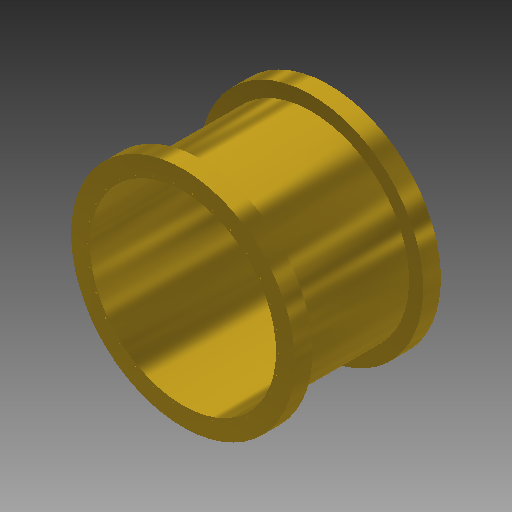
# Autodesk Inventor part: Electrode 5_6_7
Saved by Autodesk Inventor 2017 (Build 210142000, 142)
## iProperties
Created: 2009-05-06
Part Number: Electrode 5_6_7
Document SubType Name: Modeling
Designer: Serena
Material: Default
Density: 1 g/cm^3
Appearance: Glossy - Gold
Author: Serena
Autodesk Inventor part; units mm, degrees
ref_plane "YZ Plane" through (0, 0, 0) normal (1, 0, 0) x (0, 1, 0)
ref_plane "XZ Plane" through (0, 0, 0) normal (0, 1, 0) x (-1, 0, 0)
ref_plane "XY Plane" through (0, 0, 0) normal (0, 0, 1) x (1, 0, 0)
sketch "Sketch1" plane through (0, 0, 0) normal (0, 0, 1) x (1, 0, 0)
  circle A0 centre (0, 0) radius 100.35
  circle A1 centre (0, 0) radius 105.35
  dimension "d0" = 200.7
  dimension "d1" = 210.7
  constraints: 2 centre point, 1 coincident
  measures "d0" diameter of A0
  measures "d1" diameter of A1
extrude "Extrusion1" add sketch "Sketch1" along normal blind 157.48
sketch "Sketch3" plane through (0, 0, 0) normal (0, 1, 0) x (-1, 0, 0)
  line L0 (-105.35, 157.48) -> (105.35, 157.48) projected
  line L1 (-105.35, 0) -> (105.35, 0) projected
  line L2 (100.35, 0) -> (100.35, 157.48) projected
  line L3 (105.35, 0) -> (105.35, 157.48) projected
  line L4 (102.85, 157.48) -> (102.85, 55.0181)
  line L5 (102.85, 143.2846) -> (100.35, 143.2846)
  line L6 (102.85, 140.5603) -> (105.35, 140.5603)
  line L7 (102.85, 157.48) -> (102.85, 158.3207)
  circle A0 centre (102.85, 157.98) radius 1
  line L8 (102.85, 157.48) -> (102.85, 156.98)
  line L9 (102.85, 157.48) -> (103.716, 157.48)
  arc A1 (102.85, 156.98) -> (103.716, 157.48) centre (102.85, 157.98) ccw
  line L10 (102.85, 157.48) -> (102.85, 156.98)
  line L11 (102.85, 157.48) -> (103.716, 157.48)
  arc A2 (102.85, 156.98) -> (103.716, 157.48) centre (102.85, 157.98) ccw
  line L12 (102.85, 157.48) -> (102.85, 156.98)
  line L13 (102.85, 157.48) -> (101.984, 157.48)
  arc A3 (101.984, 157.48) -> (102.85, 156.98) centre (102.85, 157.98) ccw
  dimension "d15" = 2
  dimension "d16" = 0.5
  constraints: 20 end point, 9 point on circle, 9 point on line, 5 concentric, 4 centre point, 3 collinear, 3 perpendicular, 2 parallel
  measures "d15" diameter of A0
  measures "d16" distance of L4.start L8.end
revolve "Revolution1" cut sketch "Sketch3" angle 360 about axis through (-102.85, 0, 157.48) along (0, 0, -1) picked at (102.3136, 157.4236) contours L0 L4 A0
pattern_circular "Circular Pattern1" count 30 over 360 about axis through (0, 0, 0) along (0, 0, 1) of "Revolution1"
sketch "Sketch4" plane through (0, 0, 0) normal (0, 1, 0) x (-1, 0, 0)
  line L0 (-100.35, 157.48) -> (100.35, 157.48) projected
  line L1 (100.35, 0) -> (-100.35, 0) projected
  line L2 (105.35, 0) -> (105.35, 157.48) projected
  line L3 (-105.35, 0) -> (105.35, 0) projected
  line L4 (100.35, 0) -> (100.35, 157.48) projected
  line L5 (102.85, 0) -> (102.85, 39.0845)
  line L6 (102.85, 39.0845) -> (102.85, 4.4381)
  line L7 (100.35, 4.4381) -> (102.85, 4.4381)
  line L8 (102.85, 5.9556) -> (105.35, 5.9556)
  line L9 (102.85, 0) -> (102.85, -6.1846)
  circle A0 centre (102.85, -0.5) radius 1
  line L10 (102.85, 0.5) -> (102.85, 0)
  line L11 (102.85, 0) -> (103.716, 0)
  line L12 (102.85, 0) -> (101.984, 0)
  arc A1 (102.85, 0.5) -> (101.984, 0) centre (102.85, -0.5) ccw
  arc A2 (103.716, 0) -> (102.85, 0.5) centre (102.85, -0.5) ccw
  dimension "d21" = 2
  dimension "d22" = 0.5
  constraints: 16 end point, 9 point on line, 7 point on circle, 3 centre point, 3 concentric, 3 perpendicular, 2 parallel, 1 collinear
  measures "d21" diameter of A0
  measures "d22" distance of L10.start L5.start
revolve "Revolution2" cut sketch "Sketch4" angle 360 about axis through (-102.85, 0, 0.5) along (0, 0, -1) picked at (102.3136, 0.0564) contours L3 A0 L5
pattern_circular "Circular Pattern2" count 30 over 360 about axis through (0, 0, 0) along (0, 0, 1) of "Revolution2"
sketch "Sketch5" plane through (0, 0, 157.48) normal (0, 0, 1) x (1, 0, 0)
  circle A0 centre (0, 0) radius 105.35 projected
  circle A1 centre (0, 0) radius 120.65
  dimension "d27" = 241.3
  constraints: 1 centre point, 1 coincident
  measures "d27" diameter of A1
extrude "Extrusion2" add sketch "Sketch5" against normal blind 18.9992
sketch "Sketch6" plane through (0, 0, 0) normal (0, 0, -1) x (-1, 0, 0)
  circle A0 centre (0, 0) radius 105.35 projected
  circle A1 centre (0, 0) radius 120.65
  dimension "d30" = 241.3
  constraints: 1 centre point, 1 coincident
  measures "d30" diameter of A1
extrude "Extrusion3" add sketch "Sketch6" against normal blind 18.9992
equation "\"d30\" = d27"
body "Solid1"
